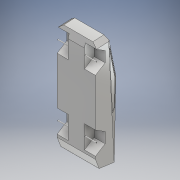
# Autodesk Inventor part: 02Cybertruck
Saved by Autodesk Inventor 2018 (Build 220112000, 112)
## iProperties
Created: 2020-06-23
Part Number: 02Cybertruck
Material: Generic
Document SubType Name: Modeling
Designer: Ivan
Density: 1 g/cm^3
Appearance: Default
Author: Ivan
Autodesk Inventor part; units mm, degrees
ref_plane "YZ Plane" through (0, 0, 0) normal (1, 0, 0) x (0, 1, 0)
ref_plane "XZ Plane" through (0, 0, 0) normal (0, 1, 0) x (-1, 0, 0)
ref_plane "XY Plane" through (0, 0, 0) normal (0, 0, 1) x (1, 0, 0)
sketch "Sketch1" plane through (0, 0, 0) normal (0, 1, 0) x (-1, 0, 0)
  line L0 (0, 0) -> (2083, 0)
  line L1 (2083, 0) -> (2083, -5885)
  line L2 (2083, -5885) -> (0, -5885)
  line L3 (0, -5885) -> (0, 0)
  dimension "d0" = 2083
  dimension "d1" = 5885
  constraints: 8 end point, 2 parallel, 1 horizontal, 1 perpendicular
  measures "d0" distance of L1.end L2.end
  measures "d1" distance of L0.end L1.end
extrude "Extrusion1" add sketch "Sketch1" along normal blind 710
sketch "Sketch2" plane through (0, 0, 0) normal (1, 0, 0) x (0, 0, -1)
  line L0 (0, 710) -> (5885, 710) projected
  line L1 (5885, 710) -> (5885, 1020)
  line L2 (5885, 710) -> (6195, 710) construction
  line L3 (5885, 1020) -> (0, 710)
  line L4 (0, 710) -> (5885, 710)
  point P0 (0, 0)
  dimension "d4" = 310
  dimension "d5" = 90
  constraints: 8 end point, 2 perpendicular, 1 horizontal, 1 vertical
  measures "d4" distance of L0.end L1.end
  measures "d5" angle of L2 L1
extrude "Extrusion2" add sketch "Sketch2" against normal up to surface (2083 mm away)
chamfer "Chamfer1" distance 420 distance2 110 1 edges at (-1041.5, 0, 0) measured on face at (-1041.5, 0, -0.5)
chamfer "Chamfer2" distance 530 distance2 200 1 edges at (-1041.5, 0, -5885) measured on face at (-1041.5, 0, -5884.5)
sketch "Sketch3" plane through (0, 110, 0) normal (1, 0, 0) x (0, 0, -1)
  line L0 (0, 600) -> (-29.9585, 598.4219)
  line L1 (5885, 910) -> (0, 600) construction
  line L2 (5885, 910) -> (5997.3442, 915.9179)
  line L3 (5885, 88.5481) -> (5885, 910)
  line L4 (5997.3442, 915.9179) -> (5885, 88.5481)
  line L5 (0, 600) -> (0, 0)
  line L6 (-29.9585, 598.4219) -> (0, 0)
  dimension "d14" = 30
  dimension "d15" = 112.5
  constraints: 12 end point, 2 collinear, 2 vertical
  measures "d14" distance of L0.start L0.end
  measures "d15" distance of L1.start L2.end
extrude "Extrusion3" add sketch "Sketch3" against normal up to surface (2083 mm away)
sketch "Sketch4" plane through (0, 0, -420) normal (1, 0, 0) x (0, 0, -1)
  line L0 (5577.3442, 1025.9179) -> (-449.9585, 708.4219) projected
  line L1 (-449.9585, 708.4219) -> (1941.6755, 1488.6146)
  line L2 (1941.6755, 1488.6146) -> (5577.3442, 1025.9179)
  line L3 (5577.3442, 1025.9179) -> (-449.9585, 708.4219)
  line L4 (1941.6755, 1488.6146) -> (1976.0415, 836.2146)
  point P0 (-420, 0)
  dimension "d20" = 2426
  dimension "d21" = 652.4
  constraints: 8 end point, 1 collinear, 1 perpendicular, 1 point on line
  measures "d20" horizontal distance of L0.end L4.end
  measures "d21" vertical distance of L1.end L4.end
extrude "Extrusion4" add sketch "Sketch4" against normal up to surface (2083 mm away)
ref_plane "Work Plane3" through (0, 708.4219, 29.9585) normal (0, -0.0499998, 0.9987492) x (1, 0, 0)
sketch "Sketch6" plane through (0, 708.4219, 29.9585) normal (0, -0.0499998, 0.9987492) x (1, 0, 0)
  line L0 (-2083, 659.6356) -> (-2083, 0) construction
  line L1 (0, 0) -> (-2083, 0) construction
  line L2 (0, 659.6356) -> (0, 0) construction
  line L3 (0, 659.6356) -> (-2083, 659.6356) construction
  line L4 (0, 0) -> (0, 659.6356)
  line L5 (0, 659.6356) -> (-380, 659.6356)
  line L6 (-380, 659.6356) -> (0, 0)
  line L7 (0, 659.6356) -> (0, 0) construction
  line L8 (-2083, 659.6356) -> (-2083, 0) construction
  line L9 (0, 0) -> (-2083, 0) construction
  line L10 (0, 0) -> (-2083, 0) projected
  line L11 (-1041.5, 0) -> (-1041.5, 659.6356) construction
  line L12 (-2083, 659.6356) -> (-2083, 0) construction
  line L13 (-2083, 0) -> (-2083, 659.6356)
  line L14 (-2083, 659.6356) -> (-1703, 659.6356)
  line L15 (-1703, 659.6356) -> (-2083, 0)
  line L16 (-2083, 659.6356) -> (-2083, 0) construction
  point P0 (0, -709.0337)
  dimension "d24" = 380
  constraints: 20 end point, 3 symmetric about line, 2 midpoint, 1 collinear, 1 horizontal, 1 point on line
  measures "d24" distance of L2.start L5.end
extrude "Extrusion5" cut sketch "Sketch6" against normal up to surface surface through (0, 1025.9179, -5997.3442) normal (0, -0.1345501, -0.9909068)
chamfer "Chamfer3" distance 250 distance2 200 1 edges at (0, 409.2109, 14.9792) measured on face at (-0.5, 409.2109, 14.9792)
chamfer "Chamfer4" distance 250 distance2 200 1 edges at (-2083, 409.2109, 14.9792) measured on face at (-2082.5, 409.2109, 14.9792)
sketch "Sketch7" plane through (-1703, 1488.6146, -2361.6755) normal (0, 0.9506933, 0.3101327) x (1, 0, 0)
  line L0 (0, 0) -> (1323, 0)
  line L1 (1323, 0) -> (1621.7173, -1977.5662)
  line L2 (1621.7173, -1977.5662) -> (-299.4539, -1977.5662)
  line L3 (-370.9356, 3312.9084) -> (0, 0) projected
  line L4 (-299.4539, -1977.5662) -> (0, 0)
  point P0 (1703, -2706.8971)
  dimension "d33" = 2000
  constraints: 8 end point, 2 horizontal
  measures "d33" distance of L0.end L1.end
extrude "Extrusion6" cut sketch "Sketch7" against normal blind 20
sketch "Sketch8" plane through (0, 718.4219, -169.7914) normal (0.8665032, 0.4985471, 0.0249585) x (0, 0.0499998, -0.9987492)
  line L0 (0, 0) -> (-22.2576, 55.7363) projected
  line L1 (5832.6944, 0) -> (0, 0) projected
  line L2 (5835.6387, 18.1589) -> (5832.6944, 0) projected
  line L3 (2227.6521, 761.2615) -> (5835.6387, 18.1589) projected
  line L4 (319.2795, 162.8353) -> (2227.6521, 761.2615) projected
  line L5 (-22.2576, 55.7363) -> (319.2795, 162.8353) projected
  line L6 (5138.8046, 80) -> (322.4868, 80)
  line L7 (322.4868, 80) -> (343.2165, 86.5004)
  line L8 (343.2165, 86.5004) -> (2231.8133, 678.7253)
  line L9 (2231.8133, 678.7253) -> (5138.8046, 80)
  line L10 (2231.8133, 678.7253) -> (3505.0878, 416.4811)
  line L11 (3505.0878, 416.4811) -> (3505.0878, 80)
  point P0 (-205.5, -614.38)
  dimension "d36" = 80
  dimension "d37" = 1300
  constraints: 12 end point, 2 point on line, 1 perpendicular, 3 other
  measures "d36" distance between parallel lines of L3 L9
  measures "d37" distance of L8.end L10.end
extrude "Extrusion7" cut sketch "Sketch8" against normal blind 20 contours L6 L7 L8 L9 L11
ref_plane "Work Plane5" through (-1041.5, 0, -420) normal (1, 0, 0) x (0, 0, -1)
mirror "Mirror1" about plane through (-1041.5, 0, -420) normal (1, 0, 0) of "Extrusion7"
sketch "Sketch9" plane through (0, 718.4219, -169.7914) normal (0.8665032, 0.4985471, 0.0249585) x (0, 0.0499998, -0.9987492)
  point P0 (-205.5, -614.38)
sketch "Sketch11" plane through (0, 0, -420) normal (1, 0, 0) x (0, 0, -1)
  line L0 (-217.089, 56.8567) -> (-250.2086, 718.4219) construction
  line L1 (-217.089, 56.8567) -> (-250.2086, 718.4219) construction
  line L2 (0, 0) -> (-217.089, 56.8567) construction
  line L3 (4935, 0) -> (0, 0) construction
  line L4 (5465, 200) -> (4935, 0) construction
  line L5 (5465, 198.5481) -> (5465, 200) construction
  line L6 (5575.1904, 1010.0556) -> (5465, 198.5481) construction
  line L7 (5575.1904, 1010.0556) -> (-250.2086, 718.4219) construction
  line L8 (-217.089, 56.8567) -> (74.3665, 523.2831)
  line L9 (-217.089, 56.8567) -> (332.911, 56.8567) construction
  line L10 (74.3665, 523.2831) -> (654.3665, 523.2831)
  line L11 (654.3665, 523.2831) -> (981.3501, 0)
  line L12 (0, 0) -> (-217.089, 56.8567) projected
  line L13 (-217.089, 56.8567) -> (0, 0)
  line L14 (0, 0) -> (981.3501, 0)
  line L15 (364.3665, 523.2831) -> (364.3665, 0) construction
  line L16 (0, 0) -> (4935, 0) construction
  line L17 (364.3665, 0) -> (4171.3665, 0) construction
  line L18 (2267.8665, 0) -> (2267.8665, 523.2831) construction
  line L19 (4788.3501, 0) -> (4461.3665, 523.2831)
  line L20 (4461.3665, 523.2831) -> (3881.3665, 523.2831)
  line L21 (3881.3665, 523.2831) -> (3554.383, 0)
  line L22 (4788.3501, 0) -> (3554.383, 0)
  point P0 (-420, 0)
  point P1 (4752.8221, 56.8567)
  dimension "d44" = 550
  dimension "d45" = 58
  dimension "d46" = 580
  dimension "d47" = 122
  dimension "d48" = 3807
  constraints: 26 end point, 5 point on line, 4 symmetric about line, 3 horizontal, 2 collinear, 2 midpoint, 1 equal length, 1 perpendicular, 1 vertical
  measures "d44" distance of L1.start L8.end
  measures "d45" angle of L9 L8
  measures "d46" distance of L8.end L10.end
  measures "d47" angle of L10 L11
  measures "d48" distance of L15.end L17.end
extrude "Extrusion9" cut sketch "Sketch11" against normal blind 600
mirror "Mirror2" about plane through (-1041.5, 0, -420) normal (1, 0, 0) of "Extrusion9"
sketch "Sketch12" plane through (0, 0, -1401.3501) normal (1, 0, 0) x (0, 0, -1)
  line L0 (-326.9836, 523.2831) -> (0, 0) construction
  line L1 (2573.0328, 0) -> (0, 0) construction
  line L2 (2573.0328, 0) -> (2900.0164, 523.2831) construction
  line L3 (2900.0164, 523.2831) -> (3480.0164, 523.2831) construction
  line L4 (3480.0164, 523.2831) -> (3807, 0) construction
  line L5 (3953.6499, 0) -> (3807, 0) construction
  line L6 (4483.6499, 200) -> (3953.6499, 0) construction
  line L7 (4483.6499, 198.5481) -> (4483.6499, 200) construction
  line L8 (4593.8403, 1010.0556) -> (4483.6499, 198.5481) construction
  line L9 (4593.8403, 1010.0556) -> (-1231.5587, 718.4219) construction
  line L10 (-1198.4392, 56.8567) -> (-1231.5587, 718.4219) construction
  line L11 (-1198.4392, 56.8567) -> (-906.9836, 523.2831) construction
  line L12 (-906.9836, 523.2831) -> (-326.9836, 523.2831) construction
  line L13 (0, 0) -> (-981.3501, 0) construction
  line L14 (-326.9836, 523.2831) -> (0, 0) construction
  line L15 (-906.9836, 523.2831) -> (-326.9836, 523.2831) construction
  line L16 (-1198.4392, 56.8567) -> (-906.9836, 523.2831) construction
  line L17 (-981.3501, 0) -> (-1198.4392, 56.8567) construction
  line L18 (-326.9836, 523.2831) -> (-906.9836, 523.2831) construction
  line L19 (-616.9836, 523.2831) -> (-616.9836, 0) construction
  line L20 (-981.3501, 0) -> (0, 0) construction
  line L21 (2573.0328, 0) -> (0, 0) construction
  line L22 (1286.5164, 0) -> (1286.5164, 696.1124) construction
  circle A0 centre (-616.9836, 50) radius 25
  circle A1 centre (3190.0164, 50) radius 25
  point P0 (-1401.3501, 0)
  dimension "d51" = 50
  dimension "d53" = 50
  constraints: 4 end point, 2 centre point, 2 midpoint, 2 point on line, 1 coincident, 1 perpendicular, 1 symmetric about line, 1 vertical, 1 other
  measures "d51" distance from line of L13 point (-616.984, 50)
  measures "d53" diameter of A0
extrude "Extrusion10" add sketch "Sketch12" against normal up to surface (600 mm away)
mirror "Mirror3" about plane through (-1041.5, 0, -420) normal (1, 0, 0) of "Extrusion10"
body "Solid1"
